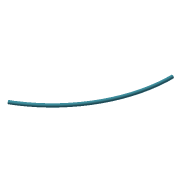
# Autodesk Inventor part: 2f2arc
Saved by Autodesk Inventor 2016 (Build 200138000, 138)
## iProperties
Company: HERA Project
Created: 2013-07-11
Part Number: 2f2arc
Material: Generic
Document SubType Name: Modeling
Designer: Dave
Density: 1 g/cm^3
Description: feed backplane pvc arc
Mass: 134.142 g
Surface Area: 939.016 cm^2
Volume: 134.142 cm^3
Appearance: Default
Author: David DeBoer
Autodesk Inventor part; units mm, degrees
ref_plane "YZ Plane" through (0, 0, 0) normal (1, 0, 0) x (0, 1, 0)
ref_plane "XZ Plane" through (0, 0, 0) normal (0, 1, 0) x (-1, 0, 0)
ref_plane "XY Plane" through (0, 0, 0) normal (0, 0, 1) x (1, 0, 0)
sketch "Sketch1" plane through (0, 0, 0) normal (0, 0, 1) x (1, 0, 0)
  circle A0 centre (596.9, -0.0117) radius 11
  line L0 (-263.1, 80.9625) -> (-263.1, -95.25)
  circle A1 centre (596.9, -0.0117) radius 9.38
  dimension "d6" = 22
  dimension "d7" = 860
  dimension "d9" = 1.62
  constraints: 2 centre point, 2 end point, 1 coincident, 1 vertical
  measures "d6" diameter of A0
  measures "d7" distance from line of L0 A0.centre
  measures "d9" radial gap between concentric circles of A1 A0
revolve "Revolution1" add sketch "Sketch1" angle 60 about axis through (-263.1, 80.9625, 0) along (0, -1, 0)
body "Solid1"
